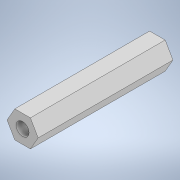
# Autodesk Inventor part: 1_2 x 2_500-inchHexShaft
Saved by Autodesk Inventor 2022.2 (Build 262287010, 287A)
## iProperties
Created: 2022-09-12
Part Number: 1_2 x 2_500-inchHexShaft
Material: Generic
Document SubType Name: Modeling
Designer: robst
Density: 1 g/cm^3
Appearance: Default
Author: robst
Autodesk Inventor part; units mm, degrees
ref_plane "YZ Plane" through (0, 0, 0) normal (1, 0, 0) x (0, 1, 0)
ref_plane "XZ Plane" through (0, 0, 0) normal (0, 1, 0) x (-1, 0, 0)
ref_plane "XY Plane" through (0, 0, 0) normal (0, 0, 1) x (1, 0, 0)
sketch "Sketch1" plane through (0, 0, 0) normal (0, 0, 1) x (1, 0, 0)
  line L0 (3.6662, 6.35) -> (7.3323, 0)
  line L1 (7.3323, 0) -> (3.6662, -6.35)
  line L2 (3.6662, -6.35) -> (-3.6662, -6.35)
  line L3 (-3.6662, -6.35) -> (-7.3323, 0)
  line L4 (-7.3323, 0) -> (-3.6662, 6.35)
  line L5 (-3.6662, 6.35) -> (3.6662, 6.35)
  circle A0 centre (0, 0) radius 2.0193
  dimension "d0" = 12.7
  dimension "d3" = 4.0386
  constraints: 12 end point, 2 coincident, 1 centre point, 1 horizontal, 13 other
  measures "d0" distance between parallel lines of L2 L5
  measures "d3" diameter of A0
extrude "Extrusion2" add sketch "Sketch1" along normal mid plane 63.5
sketch "Sketch2" plane through (0, 0, 31.75) normal (0, 0, 1) x (1, 0, 0)
  point P0 (0, 0)
  point P1 (0, 0)
  constraints: 1 coincident
hole "Hole1" at (0, 0, 31.75) direction (0, 0, -1) diameter 5.842 depth 7.874 counterbore diameter 6.096 counterbore depth 6.1239
sketch "Sketch3" plane through (0, 0, -31.75) normal (0, 0, -1) x (-1, 0, 0)
  point P0 (0, 0)
  point P1 (0, 0)
  constraints: 1 coincident
hole "Hole2" at (0, 0, -31.75) direction (0, 0, 1) diameter 5.842 depth 7.874 counterbore diameter 6.096 counterbore depth 6.1239
body "Solid2"
